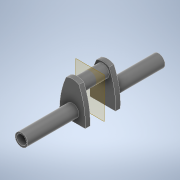
# Autodesk Inventor part: 曲轴
Saved by Autodesk Inventor 2022 (Build 260153000, 153)
## iProperties
Created: 2023-02-21
Part Number: 曲轴
Material: 常规
Document SubType Name: Modeling
Designer: 李承轩
Density: 1 g/cm^3
Appearance: 平滑 - 黑色
Author: 李承轩
Autodesk Inventor part; units mm, degrees
ref_plane "YZ Plane" through (0, 0, 0) normal (1, 0, 0) x (0, 1, 0)
ref_plane "XZ Plane" through (0, 0, 0) normal (0, 1, 0) x (-1, 0, 0)
ref_plane "XY Plane" through (0, 0, 0) normal (0, 0, 1) x (1, 0, 0)
sketch "草图1" plane through (0, 0, 0) normal (0, 0, 1) x (1, 0, 0)
  circle A0 centre (0, 0) radius 20
  dimension "d0" = 40
  constraints: 1 centre point, 1 coincident
  measures "d0" diameter of A0
extrude "拉伸1" add sketch "草图1" along normal blind 160
sketch "草图2" plane through (0, 0, 160) normal (0, 0, 1) x (1, 0, 0)
  line L0 (-40, 0) -> (40, 0)
  line L1 (40, 0) -> (40, -30) construction
  line L2 (40, -30) -> (-40, -30)
  line L3 (-40, -30) -> (-40, 0) construction
  circle A0 centre (0, 0) radius 20 projected
  line L4 (-20, 80) -> (20, 80)
  line L5 (20, 80) -> (20, -30)
  line L6 (20, -30) -> (-20, -30)
  line L7 (-20, -30) -> (-20, 80)
  line L8 (-20, 80) -> (-40, -30)
  line L9 (0, 0) -> (0, 63.2823)
  line L10 (20, 80) -> (40, -30)
  arc A1 (-20, 80) -> (-40, -30) centre (199.6341, -16.7516) ccw
  arc A2 (40, -30) -> (20, 80) centre (-199.6341, -16.7516) ccw
  arc A3 (20, 80) -> (-20, 80) centre (0, 45.359) ccw
  circle A4 centre (0, 120.4047) radius 25
  circle A5 centre (0, 0) radius 75
  line L11 (2.3516, 185.7586) -> (-119.2479, -80.6225)
  point P0 (0, -30)
  dimension "d3" = 80
  dimension "d4" = 30
  dimension "d5" = 40
  dimension "d6" = 110
  dimension "d7" = 20
  dimension "d8" = 110
  dimension "d9" = 240
  dimension "d10" = 40
  dimension "d24" = 50
  dimension "d25" = 150
  constraints: 24 end point, 6 point on circle, 5 centre point, 4 parallel, 3 midpoint, 2 coincident, 2 horizontal, 2 perpendicular, 2 tangent, 1 symmetric about line, 1 vertical, 1 vertical alignment, 1 other
  measures "d3" distance of L1.end L2.end
  measures "d4" distance of L0.end L1.end
  measures "d5" distance of L5.end L6.end
  measures "d6" distance of L4.end L5.end
  measures "d7" distance of L2.end L6.end
  measures "d8" distance of L6.end L4.start
  measures "d9" radius of A1
  measures "d10" radius of A3
  measures "d24" diameter of A4
  measures "d25" diameter of A5
extrude "拉伸2" add sketch "草图2" along normal blind 15 contours L9 A0 L0 | L0 A0 | L0 A0 L9 | L5 A5 L10 L0 | L5 L2 L7 A0 | L0 L10 L2 L5 | A0 L7 A5 L5 | L7 L2 L8 L0 | L0 L8 A5 L7 | L10 A5 A2 L0 | L0 A2 L10 | A5 L7 L4 L5 | L5 L10 A5 | L8 A1 L0 | L0 A1 A5 L8 | A5 L8 L7 | L10 A2 A5 | L4 A3 | A5 A1 L8
sketch "草图3" plane through (0, 0, 175) normal (0, 0, 1) x (1, 0, 0)
  circle A0 centre (0, 60) radius 20
  point P0 (0, 0)
  dimension "d13" = 40
  dimension "d14" = 60
  constraints: 1 centre point, 1 vertical alignment
  measures "d13" diameter of A0
  measures "d14" distance of point (0, 0) A0.centre
extrude "拉伸3" add sketch "草图3" along normal blind 80
ref_plane "工作平面1" through (0, 60, 215) normal (0, 0, 1) x (1, 0, 0)
mirror "镜像1" about plane through (0, 60, 215) normal (0, 0, 1) of "拉伸2"
mirror "镜像2" about plane through (0, 60, 215) normal (0, 0, 1) of "拉伸1"
sketch "草图4" plane through (0, 0, 430) normal (0, 0, 1) x (1, 0, 0)
  circle A0 centre (0, 0) radius 20 projected
  constraints: 1 coincident
hole "孔1" at (0, 0, 430) direction (0, 0, -1) diameter 30 depth 40
mirror "镜像3" about plane through (0, 60, 215) normal (0, 0, 1) of "孔1"
equation "\"d8\" = 5.5 * d7"
